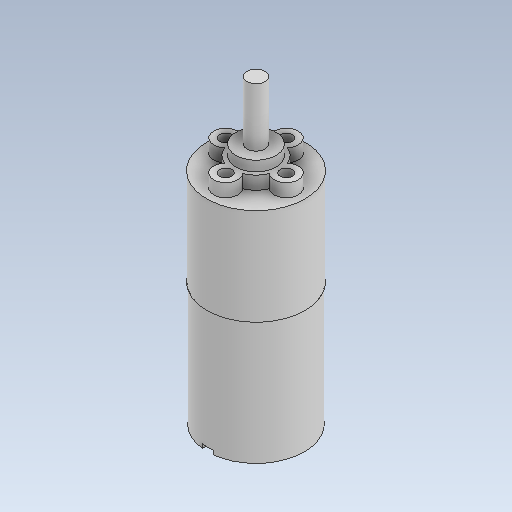
# Autodesk Inventor part: motor_2
Saved by Autodesk Inventor 2020 (Build 240168000, 168)
## iProperties
Created: 2019-04-27
Part Number: motor_2
Material: Generic
Document SubType Name: Modeling
Designer: psrob
Density: 1 g/cm^3
Appearance: Default
Author: psrob
Autodesk Inventor part; units mm, degrees
ref_plane "YZ Plane" through (0, 0, 0) normal (1, 0, 0) x (0, 1, 0)
ref_plane "XZ Plane" through (0, 0, 0) normal (0, 1, 0) x (-1, 0, 0)
ref_plane "XY Plane" through (0, 0, 0) normal (0, 0, 1) x (1, 0, 0)
sketch "Sketch1" plane through (0, 0, 0) normal (0, 1, 0) x (-1, 0, 0)
  circle A0 centre (0, 0) radius 12
  dimension "d0" = 24
  constraints: 1 centre point, 1 coincident
  measures "d0" diameter of A0
extrude "Extrusion1" add sketch "Sketch1" along normal blind 30.5
sketch "Sketch2" plane through (0, 30.5, 0) normal (0, 1, 0) x (1, 0, 0)
  circle A0 centre (0, 0) radius 12 projected
  circle A1 centre (0, 0) radius 12.2
  dimension "d3" = 24.4
  constraints: 1 centre point, 1 coincident
  measures "d3" diameter of A1
extrude "Extrusion2" add sketch "Sketch2" along normal blind 24 contours A0 | A1
sketch "Sketch3" plane through (0, 54.5, 0) normal (0, 1, 0) x (1, 0, 0)
  circle A0 centre (0, 0) radius 6
  dimension "d6" = 12
  constraints: 1 centre point, 1 coincident
  measures "d6" diameter of A0
extrude "Extrusion3" add sketch "Sketch3" along normal blind 3.25
sketch "Sketch4" plane through (0, 54.5, 0) normal (0, 1, 0) x (1, 0, 0)
  circle A0 centre (0, 0) radius 6 projected
  circle A1 centre (0, 0) radius 12.2 projected
  line L0 (0, 0) -> (-7.5, 0)
  circle A2 centre (-7.5, 0) radius 3
  circle A3 centre (0, -7.5) radius 3
  circle A4 centre (7.5, 0) radius 3
  circle A5 centre (0, 7.5) radius 3
  point P0 (-5.55, 2.2798)
  point P1 (-5.55, -2.2798)
  point P2 (2.2798, 5.55)
  point P3 (-2.2798, 5.55)
  point P4 (5.55, -2.2798)
  point P5 (5.55, 2.2798)
  point P6 (-2.2798, -5.55)
  point P7 (2.2798, -5.55)
  dimension "d9" = 7.5
  dimension "d10" = 6
  dimension "d13" = 360
  constraints: 4 centre point, 2 end point, 1 coincident, 1 horizontal, 9 other
  measures "d9" distance of L0.start L0.end
  measures "d10" diameter of A2
extrude "Extrusion4" add sketch "Sketch4" along normal blind 3.25 contours A0 A4 | A0 A5 | A3 A0 | A0 A2 picked at (7.2585, 0.8906) picked at (-1.2671, 6.9374) picked at (-1.2671, -6.9374)
sketch "Sketch5" plane through (0, 57.75, 0) normal (0, 1, 0) x (1, 0, 0)
  arc A0 (5.55, 2.2798) -> (2.2798, 5.55) centre (0, 0) ccw projected
  arc A1 (2.2798, 5.55) -> (-2.2798, 5.55) centre (0, 7.5) ccw projected
  arc A2 (-2.2798, 5.55) -> (-5.55, 2.2798) centre (0, 0) ccw projected
  arc A3 (-5.55, 2.2798) -> (-5.55, -2.2798) centre (-7.5, 0) ccw projected
  arc A4 (-5.55, -2.2798) -> (-2.2798, -5.55) centre (0, 0) ccw projected
  arc A5 (-2.2798, -5.55) -> (2.2798, -5.55) centre (0, -7.5) ccw projected
  arc A6 (2.2798, -5.55) -> (5.55, -2.2798) centre (0, 0) ccw projected
  arc A7 (5.55, -2.2798) -> (5.55, 2.2798) centre (7.5, 0) ccw projected
hole "Hole1" at (-7.5, 57.75, 0) at (0, 57.75, 7.5) at (7.5, 57.75, 0) at (0, 57.75, -7.5) direction (0, -1, 0) diameter 3 depth 5 tip angle 118
sketch "Sketch6" plane through (0, 57.75, 0) normal (0, 1, 0) x (1, 0, 0)
  circle A0 centre (0, 0) radius 5
  dimension "d24" = 10
  constraints: 1 centre point, 1 coincident
  measures "d24" diameter of A0
extrude "Extrusion5" add sketch "Sketch6" along normal blind 2.5
sketch "Sketch7" plane through (0, 60.25, 0) normal (0, 1, 0) x (1, 0, 0)
  circle A0 centre (0, 0) radius 2.25
  dimension "d27" = 4.5
  constraints: 1 centre point, 1 coincident
  measures "d27" diameter of A0
extrude "Extrusion6" add sketch "Sketch7" along normal blind 14.5
sketch "Sketch8" plane through (0, 0, 0) normal (0, -1, 0) x (1, 0, 0)
  circle A0 centre (0, 0) radius 4.125
  dimension "d30" = 8.25
  constraints: 1 centre point, 1 coincident
  measures "d30" diameter of A0
extrude "Extrusion7" add sketch "Sketch8" along normal blind 2
sketch "Sketch9" plane through (0, -2, 0) normal (0, -1, 0) x (1, 0, 0)
  circle A0 centre (0, 0) radius 4.125 projected
  circle A1 centre (0, 0) radius 1
  dimension "d33" = 2
  constraints: 1 centre point, 1 coincident
  measures "d33" diameter of A1
extrude "Extrusion8" add sketch "Sketch9" along normal blind 0.5 contours A1
sketch "Sketch10" plane through (0, 0, 0) normal (0, -1, 0) x (1, 0, 0)
  circle A0 centre (0, 0) radius 4.125 projected
  circle A1 centre (0, 0) radius 12 projected
  line L0 (0, 0) -> (0, -6.5)
  line L1 (0, 0) -> (0, 6.5)
  circle A2 centre (0, 6.5) radius 1
  circle A3 centre (0, -6.5) radius 1
  dimension "d36" = 6.5
  dimension "d37" = 6.5
  dimension "d38" = 2
  dimension "d39" = 2
  constraints: 4 end point, 2 centre point, 2 coincident, 2 vertical
  measures "d36" distance of L0.start L0.end
  measures "d37" distance of L0.start L1.end
  measures "d38" diameter of A2
  measures "d39" diameter of A3
extrude "Extrusion9" cut sketch "Sketch10" against normal blind 0.5 contours A2 | A3
sketch "Sketch11" plane through (0, 0, 0) normal (0, -1, 0) x (1, 0, 0)
  circle A0 centre (0, -6.5) radius 1 projected
  circle A1 centre (0, 6.5) radius 1 projected
  circle A2 centre (0, 0) radius 4.125 projected
  circle A3 centre (0, 0) radius 12 projected
  line L0 (0, 0) -> (0, -10.15)
  line L1 (0, 0) -> (0, 10.15)
  circle A4 centre (0, 10.15) radius 1.4
  circle A5 centre (0, -10.15) radius 1.4
  arc A6 (2.2798, 5.55) -> (-2.2798, 5.55) centre (0, 7.5) ccw projected
  line L2 (1.4, 10.1533) -> (-1.4, 10.1533)
  line L3 (-1.4, 10.1533) -> (-1.4, 13.1533)
  line L4 (-1.4, 13.1533) -> (1.4, 13.1533)
  line L5 (1.4, 13.1533) -> (1.4, 10.1533)
  arc A7 (-2.2798, -5.55) -> (2.2798, -5.55) centre (0, -7.5) ccw projected
  line L6 (1.4, -10.1533) -> (-1.4, -10.1533)
  line L7 (-1.4, -10.1533) -> (-1.4, -13.1533)
  line L8 (-1.4, -13.1533) -> (1.4, -13.1533)
  line L9 (1.4, -13.1533) -> (1.4, -10.1533)
  point P0 (-1.4, -10.1533)
  point P1 (-1.4, -11.9181)
  point P2 (1.4, -11.9181)
  point P3 (1.4, 11.9181)
  point P4 (-1.4, 11.9181)
  point P5 (-1.4, 10.1533)
  dimension "d44" = 2.8
  dimension "d45" = 2.8
  dimension "d42" = 10.15
  dimension "d43" = 10.15
  dimension "d46" = 2.8
  dimension "d47" = 3
  dimension "d48" = 2.8
  dimension "d49" = 3
  constraints: 20 end point, 4 parallel, 2 coincident, 2 horizontal, 2 perpendicular, 2 point on circle, 2 vertical, 6 other
  measures "d42" distance of L0.start L0.end
  measures "d43" distance of L0.start L1.end
  measures "d46" distance of L3.end L4.end
  measures "d47" distance of L2.end L3.end
  measures "d48" distance of L8.end L7.end
  measures "d49" distance of L7.end L6.end
extrude "Extrusion10" cut sketch "Sketch11" against normal blind 1 contours A5 L6 | A7 A5 | L6 A7 | A5 L9 A3 L7 | A3 L5 A4 L3 | A4 L2 | A4 A6 | A6 L2
sketch "Sketch12" plane through (0, 0, 0) normal (0, -1, 0) x (1, 0, 0)
  line L0 (1.4, -10.1533) -> (1.4, -11.9181) projected
  arc A0 (1.4, -11.9181) -> (1.4, 11.9181) centre (0, 0) ccw projected
  line L1 (1.4, 11.9181) -> (1.4, 10.1533) projected
  arc A1 (-1.4, 10.1533) -> (1.4, 10.1533) centre (0, 10.15) ccw projected
  line L2 (-1.4, 10.1533) -> (-1.4, 11.9181) projected
  arc A2 (-1.4, 11.9181) -> (-1.4, -11.9181) centre (0, 0) ccw projected
  line L3 (-1.4, -11.9181) -> (-1.4, -10.1533) projected
  arc A3 (1.4, -10.1533) -> (-1.4, -10.1533) centre (0, -10.15) ccw projected
  circle A4 centre (0, -6.5) radius 1 projected
  circle A5 centre (0, 6.5) radius 1 projected
  circle A6 centre (0, 0) radius 4.125 projected
  circle A7 centre (0, 0) radius 5.25
  circle A8 centre (0, 0) radius 7.5
  line L4 (0, 0) -> (7.5, 0)
  line L5 (0, 0) -> (3.75, -6.4952)
  line L6 (0, 0) -> (3.75, 6.4952)
  point P0 (2.625, 4.5466)
  point P1 (2.625, -4.5466)
  dimension "d52" = 10.5
  dimension "d53" = 15
  dimension "d54" = 60
  dimension "d55" = 60
  constraints: 6 end point, 3 point on circle, 2 centre point, 2 coincident, 1 horizontal
  measures "d52" diameter of A7
  measures "d53" diameter of A8
  measures "d54" angle of L5 L4
  measures "d55" angle of L4 L6
extrude "Extrusion11" cut sketch "Sketch12" against normal blind 0.5 contours L5 A7 L4 A8 | A8 L4 A7 L6
fillet "Fillet1" radius 1 4 edges at (3.75, 0.25, 6.4952) (2.625, 0.25, 4.5466) (2.625, 0.25, -4.5466) (3.75, 0.25, -6.4952)
pattern_circular "Circular Pattern1" count 2 over 360 about axis through (0, 0, 0) along (0, -1, 0) of "Extrusion11", "Fillet1"
body "Solid1"
